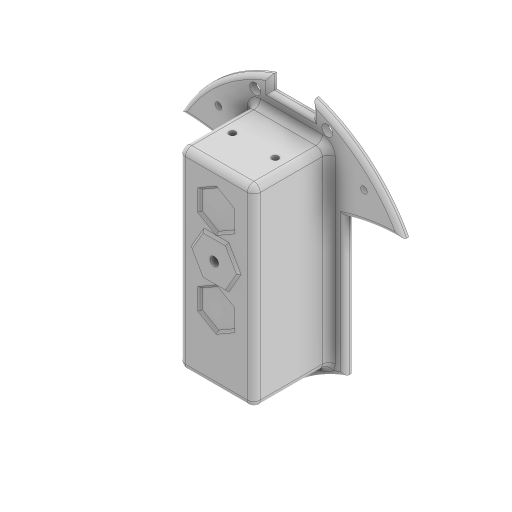
# Autodesk Inventor part: manta ray top plate
Saved by Autodesk Inventor 2024 (Build 280153000, 153)
## iProperties
Created: 2024-01-10
Part Number: manta ray top plate
Material: Generic
Document SubType Name: Modeling
Designer: chris
Density: 1 g/cm^3
Appearance: Default
Author: chris
Autodesk Inventor part; units mm, degrees
ref_plane "YZ Plane" through (0, 0, 0) normal (1, 0, 0) x (0, 1, 0)
ref_plane "XZ Plane" through (0, 0, 0) normal (0, 1, 0) x (-1, 0, 0)
ref_plane "XY Plane" through (0, 0, 0) normal (0, 0, 1) x (1, 0, 0)
sketch "Sketch2" plane through (0, 0, 0) normal (0, 0, 1) x (1, 0, 0)
  line L0 (-9.8424, 45.4565) -> (9.8424, 45.4565)
  line L1 (-9.8424, 52.2113) -> (-9.8424, 45.4565)
  arc A0 (-9.8424, 52.2113) -> (-51.9195, 16.3483) centre (14.5186, -18.9864) ccw
  arc A1 (51.9195, 16.3483) -> (9.8424, 52.2113) centre (-14.5186, -18.9864) ccw
  line L2 (9.8424, 45.4565) -> (9.8424, 52.2113)
  arc A2 (-25, 12.2891) -> (-51.9195, 16.3483) centre (-51.7248, -73.6515) ccw
  line L3 (0, 45.4565) -> (0, 56.887)
  arc A3 (51.9195, 16.3483) -> (25, 12.2891) centre (51.7248, -73.6515) ccw
  line L4 (-25, -52.7015) -> (-25, 12.2891)
  line L5 (25, -52.7015) -> (25, 12.2891)
  arc A4 (25, -52.4157) -> (0, -67.3519) centre (52.7866, -127.3149) ccw
  line L6 (0, -67.3519) -> (0, -60.3519)
  circle A5 centre (0, -60.3519) radius 1.5
  circle A6 centre (-34, 27.9565) radius 1.5
  arc A7 (0, -67.3519) -> (-25, -52.4157) centre (-52.7866, -127.3149) ccw
  circle A8 centre (34, 27.9565) radius 1.5
  point P0 (0, 0)
  point P1 (0, -30.0435)
  point P2 (14.5186, -18.9864)
  point P3 (14.5186, -18.9864)
  dimension "d0" = 90
  dimension "d2" = 7
  dimension "d3" = 3
  constraints: 14 end point, 12 point on circle, 9 centre point, 5 symmetric about line, 3 vertical, 2 point on line, 1 coincident, 1 midpoint, 1 other
  measures "d0" radius of A2
  measures "d2" distance of L6.start L6.end
  measures "d3" diameter of A5
extrude "Extrusion1" add sketch "Sketch2" along normal blind 3
fillet "Fillet1" radius 2 11 edges at (-34.2939, 38.2841, 3) (-38.3054, 15.3424, 3) (-25, -20.0633, 3) (-11.8136, -58.735, 3) (11.8136, -58.735, 3) (25, -20.0633, 3) (38.3054, 15.3424, 3) (34.2939, 38.2841, 3) (9.8424, 48.8339, 3) (0, 45.4565, 3) (-9.8424, 48.8339, 3)
sketch "Sketch3" plane through (0, 0, 3) normal (0, 0, 1) x (1, 0, 0)
  line L0 (-11.8424, 43.4565) -> (-16.8424, 43.4565)
  circle A0 centre (-16.8424, 43.4565) radius 2.5
  arc A1 (-9.8424, 52.2113) -> (-51.9195, 16.3483) centre (14.5186, -18.9864) ccw projected
  line L1 (9.8424, 45.4565) -> (-9.8424, 45.4565) projected
  line L2 (0, 45.4565) -> (0, 62.1272)
  circle A2 centre (16.8424, 43.4565) radius 2.5
  arc A3 (51.9195, 16.3483) -> (9.8424, 52.2113) centre (-14.5186, -18.9864) ccw projected
  point P0 (0, 0)
  dimension "d7" = 5
  dimension "d8" = 5
  constraints: 4 end point, 2 centre point, 1 coincident, 1 horizontal, 1 midpoint, 1 symmetric about line, 1 vertical, 1 other
  measures "d7" distance of L0.start L0.end
  measures "d8" diameter of A0
extrude "Extrusion2" cut sketch "Sketch3" against normal blind 3
sketch "Sketch4" plane through (0, 0, 3) normal (0, 0, 1) x (1, 0, 0)
  arc A0 (0, -67.3519) -> (-25, -52.4157) centre (-52.7866, -127.3149) ccw projected
  line L0 (0, -67.3519) -> (0, -52.3519)
  line L1 (0, -52.3519) -> (-17.5, -52.3519)
  line L2 (-25, 12.2891) -> (-25, -52.4157) projected
  line L3 (-17.5, -52.3519) -> (-17.5, 37.6481)
  line L4 (-17.5, 37.6481) -> (17.5, 37.6481)
  line L5 (17.5, 37.6481) -> (17.5, -52.3519)
  line L6 (17.5, -52.3519) -> (0, -52.3519)
  point P0 (0, 0)
  dimension "d12" = 15
  dimension "d13" = 17.5
  dimension "d14" = 90
  dimension "d15" = 35
  constraints: 12 end point, 5 perpendicular, 1 point on line, 1 vertical
  measures "d12" distance of L0.start L0.end
  measures "d13" distance of L0.end L1.end
  measures "d14" distance of L1.end L3.end
  measures "d15" distance of L3.end L4.end
extrude "Extrusion3" add sketch "Sketch4" along normal blind 35
sketch "Sketch5" plane through (-17.5, -52.3519, 3) normal (0, -1, 0) x (1, 0, 0)
  circle A0 centre (17.5, 17.5) radius 15.5
  point P0 (17.5, -3)
  dimension "d18" = 31
  constraints: 1 centre point
  measures "d18" diameter of A0
extrude "Extrusion4" cut sketch "Sketch5" against normal blind 87
fillet "Fillet2" radius 3 8 edges at (17.5, -52.3519, 20.5) (-17.5, -52.3519, 20.5) (17.5, 37.6481, 20.5) (-17.5, 37.6481, 20.5) (-17.5, -7.3519, 38) (0, -52.3519, 38) (17.5, -7.3519, 38) (0, 37.6481, 38)
fillet "Fillet3" radius 3 8 edges at (-16.6213, -51.4732, 3) (-17.5, -7.3519, 3) (-16.6213, 36.7694, 3) (0, 37.6481, 3) (16.6213, 36.7694, 3) (17.5, -7.3519, 3) (16.6213, -51.4732, 3) (0, -52.3519, 3)
sketch "Sketch6" plane through (0, 34.6481, 20.5) normal (0, -1, 0) x (1, 0, 0)
  line L0 (0, 0) -> (-10, 0)
  circle A0 centre (-10, 0) radius 1.5
  line L1 (0, 0) -> (10, 0)
  circle A1 centre (10, 0) radius 1.5
  point P0 (0, -20.5)
  dimension "d23" = 10
  dimension "d24" = 3
  dimension "d25" = 10
  dimension "d26" = 3
  constraints: 4 end point, 2 centre point, 2 coincident, 2 horizontal
  measures "d23" distance of L0.start L0.end
  measures "d24" diameter of A0
  measures "d25" distance of L0.start L1.end
  measures "d26" diameter of A1
extrude "Extrusion5" cut sketch "Sketch6" against normal blind 87
sketch "Sketch7" plane through (0, 0, 38) normal (0, 0, 1) x (1, 0, 0)
  line L0 (14.5, -49.3519) -> (-14.5, -49.3519) projected
  circle A0 centre (0, 0) radius 2
  dimension "d33" = 4
  constraints: 1 centre point, 1 coincident
  measures "d33" diameter of A0
extrude "Extrusion6" cut sketch "Sketch7" against normal blind 7
sketch "Sketch9" plane through (0, 0, 38) normal (0, 0, 1) x (1, 0, 0)
  circle A0 centre (0, 0) radius 2 projected
  line L0 (0, 0) -> (0, 20)
  line L1 (0, 10) -> (-8.6603, 15)
  line L2 (-8.6603, 15) -> (-8.6603, 25)
  line L3 (-8.6603, 25) -> (0, 30)
  line L4 (0, 30) -> (8.6603, 25)
  line L5 (8.6603, 25) -> (8.6603, 15)
  line L6 (8.6603, 15) -> (0, 10)
  line L7 (0, 0) -> (51.9615, 0)
  line L8 (0, 0) -> (0, -20)
  line L9 (0, -10) -> (8.6603, -15)
  line L10 (8.6603, -15) -> (8.6603, -25)
  line L11 (8.6603, -25) -> (0, -30)
  line L12 (0, -30) -> (-8.6603, -25)
  line L13 (-8.6603, -25) -> (-8.6603, -15)
  line L14 (-8.6603, -15) -> (0, -10)
  dimension "d35" = 20
  dimension "d36" = 20
  constraints: 30 end point, 2 coincident, 2 midpoint, 2 vertical, 1 horizontal, 26 other
  measures "d35" distance of L0.start L0.end
  measures "d36" distance of L0.start L8.end
extrude "Extrusion7" cut sketch "Sketch9" against normal blind 1 contours L1 L2 L3 L4 L5 L6 | L9 L10 L11 L12 L13 L14
sketch "Sketch10" plane through (0, 0, 38) normal (0, 0, 1) x (1, 0, 0)
  circle A0 centre (0, 0) radius 2 projected
  line L0 (11.547, 0) -> (5.7735, -10)
  line L1 (5.7735, -10) -> (-5.7735, -10)
  line L2 (-5.7735, -10) -> (-11.547, 0)
  line L3 (-11.547, 0) -> (-5.7735, 10)
  line L4 (-5.7735, 10) -> (5.7735, 10)
  line L5 (5.7735, 10) -> (11.547, 0)
  constraints: 12 end point, 1 coincident, 13 other
extrude "Extrusion8" add sketch "Sketch10" along normal blind 1
chamfer "Chamfer1" distance 1 angle 45 6 edges at (8.6603, 5, 39) (0, 10, 39) (-8.6603, 5, 39) (-8.6603, -5, 39) (0, -10, 39) (8.6603, -5, 39)
chamfer "Chamfer2" distance 1 angle 45 12 edges at (-4.3301, -27.5, 37) (-8.6603, -20, 37) (-4.3301, -12.5, 37) (4.3301, -27.5, 37) (8.6603, -20, 37) (4.3301, -12.5, 37) (-8.6603, 20, 37) (4.3301, 12.5, 37) (8.6603, 20, 37) (4.3301, 27.5, 37) (-4.3301, 27.5, 37) (-4.3301, 12.5, 37)
body "Solid1"
